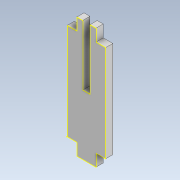
# Autodesk Inventor part: bracket
Saved by Autodesk Inventor 2022 (Build 260153000, 153)
## iProperties
Created: 2023-05-02
Part Number: bracket
Material: 一般
Document SubType Name: Modeling
Designer: JOU
Density: 1 g/cm^3
Appearance: 預設
Author: JOU
Autodesk Inventor part; units mm, degrees
ref_plane "YZ Plane" through (0, 0, 0) normal (1, 0, 0) x (0, 1, 0)
ref_plane "XZ Plane" through (0, 0, 0) normal (0, 1, 0) x (-1, 0, 0)
ref_plane "XY Plane" through (0, 0, 0) normal (0, 0, 1) x (1, 0, 0)
sketch "草圖1" plane through (0, 0, 0) normal (0, 0, 1) x (1, 0, 0)
  line L0 (0, 40) -> (16, 40)
  line L1 (16, 40) -> (16, 0)
  line L2 (16, 0) -> (0, 0)
  line L3 (0, 0) -> (0, 40)
  line L4 (4, 0) -> (12, 0)
  line L5 (12, 0) -> (12, -5)
  line L6 (12, -5) -> (4, -5)
  line L7 (4, -5) -> (4, 0)
  line L8 (4, 40) -> (12, 40)
  line L9 (12, 40) -> (12, 45)
  line L10 (12, 45) -> (4, 45)
  line L11 (4, 45) -> (4, 40)
  dimension "d0" = 16
  dimension "d1" = 5
  dimension "d2" = 8
  dimension "d3" = 4
  dimension "d4" = 40
  dimension "d5" = 5
  constraints: 24 end point, 6 parallel, 3 horizontal, 3 perpendicular, 2 collinear, 2 point on line, 1 coincident
  measures "d0" distance between parallel lines of L3 L1
  measures "d1" distance of L4.end L5.end
  measures "d2" distance between parallel lines of L7 L5
  measures "d3" distance between parallel lines of L3 L7
  measures "d4" distance of L0.end L1.end
  measures "d5" distance of L8.end L9.end
extrude "擠出1" add sketch "草圖1" along normal blind 3
sketch "草圖2" plane through (0, 0, 3) normal (0, 0, 1) x (1, 0, 0)
  line L0 (12, 45) -> (4, 45) projected
  line L1 (6.5, 45) -> (9.5, 45)
  line L2 (9.5, 45) -> (9.5, 20)
  line L3 (9.5, 20) -> (6.5, 20)
  line L4 (6.5, 20) -> (6.5, 45)
  line L5 (4, 45) -> (4, 40) projected
  point P0 (0, 0)
  dimension "d8" = 3
  dimension "d9" = 2.5
  dimension "d10" = 25
  constraints: 8 end point, 2 parallel, 1 horizontal, 1 perpendicular, 1 point on line
  measures "d8" distance between parallel lines of L4 L2
  measures "d9" distance between parallel lines of L5 L4
  measures "d10" distance of L1.end L2.end
extrude "擠出2" cut sketch "草圖2" against normal up to surface (3 mm away)
sketch "草圖3" plane through (0, 0, 3) normal (0, 0, 1) x (1, 0, 0)
  line L0 (6.5, 20) -> (6.5, 45) projected
  line L1 (6.5, 45) -> (4, 45) projected
  line L2 (4, 45) -> (4, 40) projected
  line L3 (4, 40) -> (0, 40) projected
  line L4 (0, 40) -> (0, 0) projected
  line L5 (0, 0) -> (4, 0) projected
  line L6 (4, 0) -> (4, -5) projected
  line L7 (4, -5) -> (12, -5) projected
  line L8 (12, -5) -> (12, 0) projected
  line L9 (12, 0) -> (16, 0) projected
  line L10 (16, 0) -> (16, 40) projected
  line L11 (16, 40) -> (12, 40) projected
  line L12 (12, 40) -> (12, 45) projected
  line L13 (12, 45) -> (9.5, 45) projected
  line L14 (9.5, 45) -> (9.5, 20) projected
  line L15 (9.5, 20) -> (6.5, 20) projected
